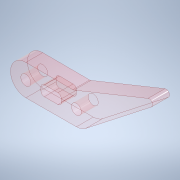
# Autodesk Inventor part: カウンター 先端部
Saved by Autodesk Inventor 2020.2 (Build 242310000, 310)
## iProperties
Created: 2020-05-03
Part Number: カウンター 先端部
Material: ポリカーボネート、クリア
Document SubType Name: Modeling
Designer: mozar
Density: 1.2 g/cm^3
Appearance: 透明 - 淡い赤
Mass: 1.67314 g
Surface Area: 12.4751 cm^2
Volume: 1.39428 cm^3
Author: mozar
Autodesk Inventor part; units mm, degrees
ref_plane "YZ Plane" through (0, 0, 0) normal (1, 0, 0) x (0, 1, 0)
ref_plane "XZ Plane" through (0, 0, 0) normal (0, 1, 0) x (-1, 0, 0)
ref_plane "XY Plane" through (0, 0, 0) normal (0, 0, 1) x (1, 0, 0)
sketch "スケッチ1" plane through (0, 0, 0) normal (0, 0, 1) x (1, 0, 0)
  circle A0 centre (132.465, 0) radius 1.5
  circle A1 centre (45, 0) radius 1.5
  circle A2 centre (102.465, 0) radius 1.5
  circle A3 centre (72.465, 0) radius 1.5
  circle A4 centre (15, 0) radius 1.5
  circle A5 centre (30, 0) radius 1.5
  circle A6 centre (87.465, 0) radius 1.5
  circle A7 centre (117.465, 0) radius 1.5
  circle A8 centre (60, 0) radius 1.5
  circle A9 centre (0, 0) radius 1.5
  line L0 (132.482, -4.5) -> (0.0189, -5)
  arc A10 (0.0189, 5) -> (0.0189, -5) centre (0, 0) ccw
  line L1 (0.0189, 5) -> (132.482, 4.5)
  arc A11 (132.482, -4.5) -> (132.482, 4.5) centre (132.465, 0) ccw
  circle A12 centre (117.465, 0) radius 4.5566
  line L2 (135.2384, -3.5437) -> (160.3015, 16.0714)
  circle A13 centre (132.465, 0) radius 4.5
  line L3 (130.7828, 4.1737) -> (160.3015, 16.0714)
  circle A14 centre (154.1156, 12.5) radius 1
  point P0 (117.4822, -4.5566)
  point P1 (154.732, 11.7125)
  point P2 (153.7418, 13.4275)
  point P3 (131.6004, 4.5033)
  point P4 (117.4822, 4.5566)
  dimension "d0" = 2
  dimension "d1" = 25
  dimension "d2" = 150
  constraints: 15 centre point, 8 end point, 7 point on circle, 5 tangent, 2 coincident, 32 other
  measures "d0" diameter of A14
  measures "d1" distance of A0.centre A14.centre
extrude "押し出し1" add sketch "スケッチ1" against normal blind 5 contours A13 A11 | L0 A12 L1 L3 A13 | A12 | A11 L1 L3 A14 L2 | L3 L1 A13 | A14
fillet "フィレット1" radius 1 1 edges at (131.6004, 4.5033, -2.5)
sketch "スケッチ2" plane through (0, 0, 0) normal (0, 0, 1) x (1, 0, 0)
  circle A0 centre (117.465, 0) radius 1.5 projected
  circle A1 centre (132.465, 0) radius 1.5 projected
  line L0 (132.482, -4.5) -> (117.4822, -4.5566) projected
  arc A2 (117.4822, 4.5566) -> (117.4822, -4.5566) centre (117.465, 0) ccw projected
  line L1 (117.4822, 4.5566) -> (131.4045, 4.504) projected
  arc A3 (131.4045, 4.504) -> (131.7821, 4.5765) centre (131.4083, 5.504) ccw projected
  line L2 (131.7821, 4.5765) -> (153.7418, 13.4275) projected
  arc A4 (154.732, 11.7125) -> (153.7418, 13.4275) centre (154.1156, 12.5) ccw projected
  line L3 (154.732, 11.7125) -> (135.2384, -3.5437) projected
  arc A5 (132.482, -4.5) -> (135.2384, -3.5437) centre (132.465, 0) ccw projected
  line L4 (131.3932, 1.5041) -> (117.4709, 1.5566)
  arc A6 (117.4709, 1.5566) -> (117.4709, -1.5566) centre (117.465, 0) ccw
  line L5 (117.4709, -1.5566) -> (132.4707, -1.5)
  arc A7 (132.4707, -1.5) -> (133.3895, -1.1812) centre (132.465, 0) ccw
  line L6 (133.3895, -1.1812) -> (141.7438, 5.3571)
  line L7 (141.7438, 5.3571) -> (132.9036, 1.794)
  arc A8 (131.3932, 1.5041) -> (132.9036, 1.794) centre (131.4083, 5.504) ccw
  circle A9 centre (117.465, 0) radius 4.5
  circle A10 centre (132.465, 0) radius 4.5
  circle A11 centre (136.965, 2.8567) radius 1
  point P0 (0, 0)
  point P1 (128.2281, -1.516)
  point P2 (128.2281, 1.516)
  point P3 (121.693, 1.5407)
  point P4 (121.693, -1.5407)
  dimension "d6" = 3
  dimension "d7" = 3
  dimension "d8" = 3
  dimension "d9" = 2
  constraints: 8 end point, 6 centre point, 6 point on circle, 6 other
  measures "d6" distance between parallel lines of L1 L4
  measures "d7" radial gap between concentric circles of A0 A9
  measures "d8" radial gap between concentric circles of A1 A10
  measures "d9" diameter of A11
extrude "押し出し2" cut sketch "スケッチ2" against normal blind 4.5 contours L5 A9 L4 A10
fillet "フィレット2" radius 1 4 edges at (121.693, 1.5407, -2.25) (121.693, -1.5407, -2.25) (128.2281, 1.516, -2.25) (128.2281, -1.516, -2.25)
